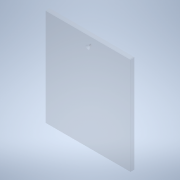
# Autodesk Inventor part: J001843
Saved by Autodesk Inventor 2020.3 (Build 243373000, 373)
## iProperties
RuleStatus: InUse
AfterDocSave0: file://Part Number Cleaner
Created: 2012-08-06
Part Number: J001843
Material: GLASS, BOROSILICATE
Vendor: HHMI: JFRC - ID&F
Document SubType Name: Modeling
Designer: NEGRASHOVI
Mass: 262.504 g
Surface Area: 406.059 cm^2
Volume: 117.715 cm^3
Density: 2.23 g/cm^3
Project: P-75301
Description: CHAMBER COVER GLASS
Appearance: Clear - Light
LAB/DEPT: RUBIN (LAB)
REQUESTING SCIENTIST: ASO, YOSHI
SURFACE ROUGHNESS: N/A
DESIGN DEPARTMENT: HHMI: JRC - ID&F
SPECIAL FINISH: NONE
ALTERED ITEM PART NUMBER: N/A
ALTERED ITEM VENDOR: N/A
ALTERED ITEM DESCRIPTION: N/A
Author: NEGRASHOVI
Revision Number: B
Autodesk Inventor part; units mm, degrees
ref_plane "YZ Plane" through (0, 0, 0) normal (1, 0, 0) x (0, 1, 0)
ref_plane "XZ Plane" through (0, 0, 0) normal (0, 1, 0) x (-1, 0, 0)
ref_plane "XY Plane" through (0, 0, 0) normal (0, 0, 1) x (1, 0, 0)
sketch "Sketch1" plane through (0, 0, 0) normal (0, 0, 1) x (1, 0, 0)
  line L0 (-63.5, 73.025) -> (63.5, 73.025)
  line L1 (63.5, 73.025) -> (63.5, -73.025)
  line L2 (63.5, -73.025) -> (-63.5, -73.025)
  line L3 (-63.5, -73.025) -> (-63.5, 73.025)
  point P0 (0, 0)
  dimension "d0" = 127
  dimension "d1" = 146.05
  dimension "d2" = 73.025
  dimension "d3" = 63.5
  constraints: 8 end point, 2 parallel, 1 horizontal, 1 perpendicular
  measures "d0" distance of L0.start L0.end
  measures "d1" distance of L2.end L0.start
  measures "d2" distance from line of point (0, 0) L0
  measures "d3" distance from line of point (0, 0) L3
extrude "Extrusion1" add sketch "Sketch1" along normal blind 6.35
sketch "Sketch2" plane through (0, 0, 6.35) normal (0, 0, 1) x (1, 0, 0)
  line L0 (0, -102.235) -> (0, 102.235) construction
  line L1 (-63.5, 73.025) -> (63.5, 73.025) projected
  line L2 (-63.5, -73.025) -> (-63.5, 73.025) projected
  line L3 (63.5, 73.025) -> (63.5, -73.025) projected
  line L4 (63.5, -73.025) -> (-63.5, -73.025) projected
  line L5 (63.5, 73.025) -> (63.5, -73.025) projected
  line L6 (-63.5, 73.025) -> (63.5, 73.025) projected
  line L7 (-63.5, -73.025) -> (-63.5, 73.025) projected
  line L8 (63.5, -73.025) -> (-63.5, -73.025) projected
  circle A0 centre (0, -6.35) radius 50.8 construction
  point P0 (0, 0)
  point P1 (0, 57.15)
  point P2 (0, -57.15)
  point P3 (-38.1, -39.951)
  point P4 (38.1, -39.951)
  dimension "d15" = 15.875
  dimension "d16" = 15.875
  dimension "d17" = 101.6
  dimension "d18" = 76.2
  constraints: 3 point on circle, 3 point on line, 1 centre point, 1 symmetric about line
  measures "d15" distance from line of point (0, 57.15) L1
  measures "d16" distance from line of A0.start L4
  measures "d17" diameter of A0
  measures "d18" distance of point (38.1, -39.951) A0.end
hole "Hole1" at (0, 57.15, 6.35) direction (0, 0, -1) diameter 3.175 end through all countersink diameter 6.35 countersink angle 90
chamfer "Chamfer1" distance 0.8128 angle 45 12 edges at (0, 73.025, 6.35) (-63.5, 0, 6.35) (63.5, 0, 6.35) (0, -73.025, 6.35) (63.5, 73.025, 3.175) (63.5, -73.025, 3.175) (-63.5, 73.025, 3.175) (-63.5, -73.025, 3.175) (-63.5, 0, 0) (0, 73.025, 0) (63.5, 0, 0) (0, -73.025, 0)
equation "\"d2\" = 0.5 * d1"
equation "\"d3\" = 0.5 * d0"
equation "\"d16\" = d15"
body "Solid1"
